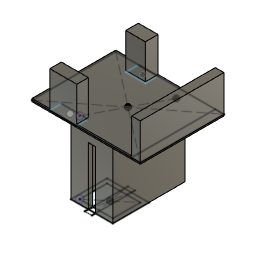
motor_hold v5 (Autodesk Fusion 360 design; units mm, degrees)
Autodesk Fusion 360 part; units mm, degrees
sketch "Sketch1" plane through (0, 0, 0) normal (0, 0, 1) x (1, 0, 0)
  line L0 (0, 0) -> (23, 0)
  line L1 (23, 0) -> (23, 19)
  line L2 (23, 19) -> (0, 19)
  line L3 (0, 19) -> (0, 0)
  line L4 (0, 0) -> (23, 19) construction
  line L5 (14, -5.5) -> (9, -5.5) construction
  line L6 (9, -5.5) -> (9, 24.5)
  line L7 (9, 24.5) -> (14, 24.5) construction
  line L8 (14, 24.5) -> (14, -5.5)
  line L9 (14, -5.5) -> (9, 24.5) construction
  line L10 (9, -5.5) -> (14, 24.5) construction
  line L11 (-3, 22) -> (-3, -3)
  line L12 (-3, -3) -> (26, -3)
  line L13 (26, -3) -> (26, 22)
  line L14 (26, 22) -> (-3, 22)
  point P0 (11.5, 9.5)
  dimension "d1" = 23
  dimension "d2" = 19
  dimension "d5" = 5
  dimension "d6" = 3
  dimension "d11" = 30
  constraint horizontal L0
  constraint vertical L1
  constraint horizontal L2
  constraint vertical L3
  constraint coincident L0.start L3.end
  constraint horizontal L5
  constraint perpendicular L5 L6
  constraint parallel L5 L7
  constraint parallel L6 L8
  constraint coincident L9 P0
  constraint coincident L10 P0
  constraint midpoint L4 P0
  measures "d1" distance of L0.start L0.end
  measures "d2" distance of L0.start L2.end
  measures "d5" distance of L6.end L7.end
  measures "d11" distance of L5.end L6.end
extrude "Extrude4" add sketch "Sketch1" along normal blind 50 contours L0 L2 L3 L6 L11 L12 L14 | L0 L1 L2 L8 L12 L13 L14 makes body 1 at (-3, 13.6667, 16.6667) makes body 2 at (26, 5.3333, 16.6667)
sketch "Sketch2" plane through (0, 0, 50) normal (0, 0, 1) x (-1, 0, 0)
  line L0 (-14, 0) -> (-14, 3)
  line L1 (-14, 3) -> (-26, 3)
  line L2 (-26, 3) -> (-26, -22)
  line L3 (-26, -22) -> (-14, -22)
  line L4 (-14, -22) -> (-14, -19)
  line L5 (-14, -19) -> (-23, -19)
  line L6 (-23, -19) -> (-23, 0)
  line L7 (-23, 0) -> (-14, 0)
  line L8 (0.208, -22.1542) -> (-23, -22.1542)
  line L9 (-23, -22.1542) -> (-23, -19)
  line L10 (-23, -19) -> (0.208, -19)
  line L11 (0.208, -19) -> (0.208, -22.1542)
  line L12 (0, 0) -> (-23, 0)
  line L13 (-23, 0) -> (-23, 3)
  line L14 (-23, 3) -> (0, 3)
  line L15 (0, 3) -> (0, 0)
  constraint horizontal L8
  constraint vertical L9
  constraint horizontal L10
  constraint vertical L11
  constraint coincident L5.end L6.start
  constraint horizontal L12
  constraint vertical L13
  constraint horizontal L14
  constraint vertical L15
  constraint coincident L1 L13.end
  constraint coincident L12.start L15.end
extrude "Extrude5" add sketch "Sketch2" against normal blind 10 contours L0 L1 L7 L12 L13 L14 | L0 L12 L14 L15 | L3 L4 L5 L9 L10 | L3 L4 L8 L9 L10 L11 bodies 1 2
copy_body "CopyPasteBodies1" bodies 1 makes body 3
move_body "Move1" bodies 3 to x (1, 0, 0) y (0, 1, 0) z (0, 0, 1) at (0, 30, 0)
move_body "Move2" bodies 3 to x (1, 0, 0) y (0, 1, 0) z (0, 0, 1) at (0, -5, 0)
sketch "Sketch3" plane through (0, 0, 50) normal (0, 0, 1) x (-1, 0, 0)
  line L0 (0, -44) -> (-23, -44)
  line L1 (-23, -44) -> (-23, -25)
  line L2 (-23, -25) -> (0, -25)
  line L3 (0, -25) -> (0, -44)
  line L4 (-23, -47) -> (-23, -47.1542)
  line L5 (-23, -47.1542) -> (0.208, -47.1542)
  line L6 (0.208, -47.1542) -> (0.208, -47)
  line L7 (0.208, -47) -> (3, -47)
  line L8 (3, -47) -> (3, -22)
  line L9 (3, -22) -> (-26, -22)
  line L10 (-26, -22) -> (-26, -47)
  line L11 (-26, -47) -> (-23, -47)
  line L12 (0, 0) -> (-23, -44) construction
  line L13 (26, 7) -> (-49, 7)
  line L14 (-49, 7) -> (-49, -51)
  line L15 (-49, -51) -> (26, -51)
  line L16 (26, -51) -> (26, 7)
  line L17 (26, 7) -> (-49, -51) construction
  line L18 (-49, 7) -> (26, -51) construction
  line L19 (-49, -51) -> (-43, -51) construction
  line L20 (-43, -51) -> (-43, 7)
  line L21 (13.676, 7) -> (-5, 7)
  line L22 (-5, 7) -> (-5, -1)
  line L23 (-5, -1) -> (13.676, -1)
  line L24 (13.676, -1) -> (13.676, 7)
  line L25 (10.3139, -51) -> (-3.2871, -51)
  line L26 (-3.2871, -51) -> (-3.2871, -42.2509)
  line L27 (-3.2871, -42.2509) -> (10.3139, -42.2509)
  line L28 (10.3139, -42.2509) -> (10.3139, -51)
  point P0 (-11.5, -22)
  point P1 (3, -46.6655)
  point P2 (4.6174, 2.0386)
  dimension "d16" = 75
  dimension "d17" = 58
  dimension "d22" = 6
  dimension "d23" = 8
  constraint coincident L12.start origin
  constraint coincident L0.end L1.start
  constraint horizontal L13
  constraint perpendicular L13 L14
  constraint parallel L13 L15
  constraint parallel L14 L16
  constraint coincident L17 P0
  constraint coincident L18 P0
  constraint midpoint L12 P0
  constraint perpendicular L14 L19
  constraint coincident L13 L20.end
  constraint perpendicular L13 L20
  constraint coincident L8 P1
  constraint horizontal L21
  constraint vertical L22
  constraint horizontal L23
  constraint vertical L24
  constraint coincident L13 L21.start
  constraint horizontal L25
  constraint vertical L26
  constraint horizontal L27
  constraint vertical L28
  constraint coincident L15 L25.start
  measures "d16" distance of L14.end L15.end
  measures "d17" distance of L13.end L14.end
  measures "d22" distance of L14.end L19.end
  measures "d23" distance of L21.start L23.end
extrude "Extrude6" add sketch "Sketch3" along normal blind 1 and the other way blind 1 bodies 1 3
extrude "Extrude7" add sketch "Sketch3" along normal blind 25 contours L0 L3 L5 L6 L7 L8 L26 L27 | L0 L3 L26 L27 | L5 L6 L7 L8 L15 L25 L26 L27 L28 | L13 L14 L15 L20 | L13 L21 L22 L23 L24 bodies 1
